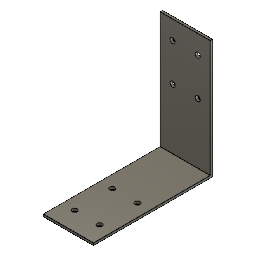
09part (Autodesk Fusion 360 design; units mm, degrees)
Autodesk Fusion 360 part; units mm, degrees
sketch "Sketch1" plane through (0, 0, 0) normal (0, 0, 1) x (1, 0, 0)
  line L0 (-20, 95) -> (20, 95)
  line L1 (20, 95) -> (20, 0)
  line L2 (20, 0) -> (-20, 0)
  line L3 (-20, 0) -> (-20, 95)
  circle A0 centre (-10, 80) radius 2
  circle A1 centre (10, 80) radius 2
  circle A2 centre (-10, 50) radius 2
  circle A3 centre (10, 50) radius 2
  line L4 (0, 125) -> (0, -25) construction
  dimension "d1" = 95
  dimension "d2" = 40
  dimension "d3" = 4
  dimension "d8" = 20
  dimension "d9" = -30
  dimension "d10" = 15
  constraint horizontal L0
  constraint vertical L1
  constraint horizontal L2
  constraint vertical L3
  constraint midpoint origin L2
  constraint vertical L4
  constraint coincident origin L4
  constraint symmetric A0.centre A1.centre L4
  measures "d1" distance of L0.start L2.end
  measures "d2" distance of L0.start L0.end
  measures "d3" diameter of A0
  measures "d10" distance of L0 A1.centre
extrude "Extrude1" add sketch "Sketch1" along normal blind 2 makes body 1
ref_plane "WorkPlane1" through (0, 0, 0) normal (0, 0.707107, -0.707107) x (-1, 0, 0)
mirror "Mirror1" about plane through (0, 0, 0) normal (0, 0.707107, -0.707107) of "Extrude1" makes body 2
combine "Combine1" operation add target body 2 tool bodies 1
